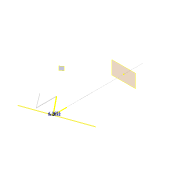
# Autodesk Inventor part: 00_Beampath_v0
Saved by Autodesk Inventor 2022 (Build 260153000, 153)
## iProperties
Created: 2022-04-09
Part Number: 00_Beampath_v0
Material: Generic
Document SubType Name: Modeling
Designer: Prakash Lab
Density: 1 g/cm^3
Appearance: Default
Author: Prakash Lab
Autodesk Inventor part; units mm, degrees
ref_plane "YZ Plane" through (0, 0, 0) normal (1, 0, 0) x (0, 1, 0)
ref_plane "XZ Plane" through (0, 0, 0) normal (0, 1, 0) x (-1, 0, 0)
ref_plane "XY Plane" through (0, 0, 0) normal (0, 0, 1) x (1, 0, 0)
ref_plane "Work Plane1" through (0, 0, 0) normal (0, 0, 1) x (1, 0, 0)
sketch "Sketch1" plane through (0, 0, 0) normal (0, 0, 1) x (1, 0, 0)
  circle A0 centre (0, 0) radius 0.5
  dimension "d0" = 1
  constraints: 1 centre point, 1 coincident
  measures "d0" diameter of A0
extrude "Extrusion1" add sketch "Sketch1" along normal blind 170 and the other way blind 105
sketch "Sketch2" plane through (0, 0, 170) normal (0, 0, 1) x (1, 0, 0)
  circle A0 centre (0, 0) radius 0.5
  circle A1 centre (0, 0) radius 0.820825
  constraints: 1 centre point, 1 coincident
extrude "Extrusion2" add sketch "Sketch2" along normal blind 75 contours A0 | A1
sketch "Sketch3" plane through (0, 0, 245) normal (0, 0, 1) x (1, 0, 0)
  circle A0 centre (0, 0) radius 0.820825
  circle A1 centre (0, 0) radius 0.5
  circle A2 centre (0, 0) radius 0.5
  constraints: 1 centre point, 1 coincident
extrude "Extrusion3" add sketch "Sketch3" along normal blind 75 contours A1
sketch "Sketch4" plane through (0, 0, 320) normal (0, 0, 1) x (1, 0, 0)
  circle A0 centre (0, 0) radius 0.820825
extrude "Extrusion4" add sketch "Sketch4" along normal blind 75
sketch "Sketch5" plane through (0, 0, 0) normal (0, 1, 0) x (-1, 0, 0)
  line L0 (-0.820825, 320) -> (-0.820825, 395)
  line L1 (-0.820825, 320) -> (-0.820825, 395)
  line L2 (0.820825, 320) -> (0.820825, 395)
  line L3 (0.820825, 395) -> (-0.820825, 395)
  line L4 (0, 395) -> (201.982812, 145.572)
  line L5 (0, 395) -> (-0.820825, 394.335309)
  line L6 (-0.820825, 394.335309) -> (80.573337, 293.82189)
  line L7 (80.573337, 293.82189) -> (81.394162, 294.486581)
  point P0 (0, 0)
  point P1 (0.820825, 393.986366)
  point P2 (0.820825, 392.308042)
  dimension "d11" = 39
  dimension "d12" = 249.428
  constraints: 8 end point, 2 point on line, 1 midpoint, 1 parallel, 1 perpendicular
  measures "d11" angle of L0 L4
  measures "d12" vertical distance of L4.start L4.end
ref_plane "Work Plane2" through (-201.982812, 0, 145.572) normal (-0.6293204, 0, -0.777146) x (0, -1, 0)
revolve "Revolution1" add sketch "Sketch5" angle 360 about axis through (0, 0, 395) along (-0.6293204, 0, -0.777146) contours L5 L4 L2 L6 | L2 L4 L7 L6
sketch "Sketch10" plane through (0, 0, 0) normal (0, 1, 0) x (-1, 0, 0)
  line L0 (82.214986, 295.151272) -> (80.573337, 293.82189)
  line L1 (82.214986, 295.151272) -> (80.573337, 293.82189)
  line L2 (81.394162, 294.486581) -> (81.394162, 406.830692)
  line L3 (82.214986, 295.151272) -> (79.881571, 295.151272)
  line L4 (79.881571, 295.151272) -> (79.881571, 406.830692)
  line L5 (79.881571, 406.830692) -> (81.394162, 406.830692)
  line L6 (82.214986, 295.151272) -> (0.820825, 395.664691)
  point P0 (0, 0)
  point P1 (2.462474, 393.637423)
  point P2 (79.881571, 298.0328)
  point P3 (81.394162, 296.164905)
  point P4 (81.394162, 295.151272)
  dimension "d18" = 39
  constraints: 8 end point, 2 perpendicular, 1 midpoint, 1 parallel
  measures "d18" angle of L6 L2
revolve "Revolution2" add sketch "Sketch10" angle 360 about axis through (-81.394162, 0, 294.486581) along (0, 0, 1) contours L3 L4 L6 L2 | L6 L4 L5 L2
sketch "Sketch11" plane through (0, 0, 0) normal (0, 1, 0) x (-1, 0, 0)
  line L0 (79.881571, 298.0328) -> (79.881571, 406.830692)
  line L1 (82.906753, 295.151272) -> (82.906753, 406.830692)
  line L2 (82.906753, 406.830692) -> (79.881571, 406.830692)
  line L3 (81.394162, 406.830692) -> (140.440427, 328.159447)
  line L4 (140.440427, 328.159447) -> (139.422813, 327.395682)
  line L5 (139.422813, 327.395682) -> (80.376547, 406.066927)
  line L6 (80.376547, 406.066927) -> (81.394162, 406.830692)
  point P0 (0, 0)
  constraints: 8 end point, 3 perpendicular, 1 midpoint, 1 point on line
revolve "Revolution3" add sketch "Sketch11" angle 360 about axis through (-81.394162, 0, 406.830692) along (-0.6002786, 0, -0.7997909) contours L5 L6 L3 L1 | L1 L3 L4 L5
sketch "Sketch12" plane through (0, 0, 0) normal (0, 1, 0) x (-1, 0, 0)
  line L0 (82.214986, 295.151272) -> (80.573337, 293.82189)
  line L1 (82.214986, 295.151272) -> (80.196137, 295.151272)
  line L2 (80.196137, 295.151272) -> (82.214986, 295.151272)
  line L3 (0.820825, 320) -> (-0.820825, 320)
  line L4 (4.715038, 389.177413) -> (-3.452339, 399.263283)
  line L5 (0, 383.095672) -> (0, 396.614396)
  line L6 (-2.252032, 394.202514) -> (2.252032, 395.797486)
  line L7 (79.881571, 298.0328) -> (0.820825, 395.664691)
  line L8 (-0.820825, 320) -> (-0.820825, 394.335309)
  line L9 (0.820825, 320) -> (0.820825, 392.308042)
  line L10 (80.573337, 293.82189) -> (0.820825, 392.308042)
  line L11 (-0.820825, 394.335309) -> (0, 395)
  line L12 (0, 395) -> (-0.820825, 394.335309)
  point P0 (0, 0)
  point P1 (0.820825, 392.308042)
  point P2 (2.462474, 393.637423)
  point P3 (0.820825, 392.308042)
  point P4 (0.820825, 393.986366)
  point P5 (0.820825, 395)
  point P6 (-0.820825, 395)
  point P7 (0, 395)
  dimension "d21" = 1.64165
  dimension "d22" = 0.82082
  constraints: 6 end point, 1 midpoint, 1 parallel, 1 vertical, 3 other
  measures "d21" distance between parallel lines of L9 L8
  measures "d22" distance between parallel lines of L8 L5
ref_plane "Work Plane5" through (0, 0, 395) normal (0.3338069, 0, 0.9426415) x (0, 1, 0)
sketch "Sketch13" plane through (0, 0, 395) normal (0.3338069, 0, 0.9426415) x (0, 1, 0)
  ellipse E0 centre (0, 0) end of major axis (1.056204, 0) minor radius 0.995622
  circle A0 centre (0, 0) radius 1.898257
  point P0 (0, -131.853709)
  point P1 (0, -0.995622)
  constraints: 1 centre point, 1 coincident, 1 vertical alignment
extrude "Extrusion7" cut sketch "Sketch13" along normal blind 25.4 contours E0 | A0
sketch "Sketch14" plane through (0, 0, 395) normal (0.3338069, 0, 0.9426415) x (0.9426415, 0, -0.3338069)
  ellipse E0 centre (0, 0) end of major axis (1.120472, 0) minor radius 1.056204 (0, 1.056204) -> (0, -1.056204) ccw
  line L0 (0, -0.820825) -> (0, -1.056204)
  ellipse E1 centre (0, 0) end of major axis (0.870771, 0) minor radius 0.820825 (0, -0.820825) -> (0, 0.820825) ccw
  line L1 (0, 1.056204) -> (0, 0.820825)
  circle A0 centre (0, 0) radius 0.310652
  point P0 (131.853709, 0)
  constraints: 1 centre point, 1 coincident, 2 other
extrude "Extrusion8" cut sketch "Sketch14" against normal blind 25.4 contours A0
sketch "Sketch15" plane through (0, 0, 0) normal (0, 1, 0) x (-1, 0, 0)
  line L0 (79.881571, 298.0328) -> (79.881571, 406.830692)
  line L1 (82.906753, 295.151272) -> (82.906753, 402.695767)
  line L2 (75.780569, 301.41879) -> (84.581608, 290.550413)
  line L3 (81.394162, 304.987675) -> (81.394162, 291.424331)
  line L4 (80.573337, 293.82189) -> (0.820825, 392.308042)
  line L5 (79.881571, 298.0328) -> (0.820825, 395.664691)
  line L6 (76.652956, 292.807632) -> (85.693899, 296.009198)
  line L7 (79.881571, 293.950944) -> (83.678666, 295.295566)
  line L8 (83.678666, 295.295566) -> (83.56271, 295.623018)
  line L9 (83.56271, 295.623018) -> (79.765614, 294.278396)
  line L10 (79.765614, 294.278396) -> (79.881571, 293.950944)
  line L11 (82.756792, 406.830692) -> (82.756792, 406.830692)
  line L12 (80.196137, 295.151272) -> (80.196137, 295.151272)
  line L13 (82.756792, 406.830692) -> (81.394162, 406.830692)
  line L14 (81.394162, 406.830692) -> (82.756792, 406.830692)
  line L15 (81.394162, 406.830692) -> (81.394162, 406.830692)
  line L16 (141.458041, 328.923212) -> (139.422813, 327.395682)
  line L17 (139.422813, 327.395682) -> (82.906753, 402.695767)
  line L18 (141.458041, 328.923212) -> (82.411776, 407.594457)
  line L19 (79.881571, 298.0328) -> (79.881571, 406.830692)
  line L20 (82.906753, 295.151272) -> (82.906753, 402.695767)
  line L21 (81.394162, 394.279852) -> (81.394162, 413.621168)
  line L22 (86.59775, 399.897607) -> (77.597609, 411.889091)
  line L23 (78.065498, 405.720493) -> (84.224665, 407.774741)
  line L24 (84.224665, 407.774741) -> (84.614224, 406.606742)
  line L25 (84.614224, 406.606742) -> (78.455057, 404.552494)
  line L26 (78.455057, 404.552494) -> (78.065498, 405.720493)
  point P0 (0, 0)
  point P1 (81.394162, 294.486581)
  dimension "d27" = 2.11241
  dimension "d28" = 3.02518
  dimension "d29" = 1.0562
  dimension "d30" = 1.51259
  dimension "d31" = 39
  dimension "d32" = 109.5
  dimension "d38" = 36.8899
  dimension "d39" = 71.5551
  dimension "d40" = 1.51259
  dimension "d41" = 2.5447
  dimension "d42" = 1.27235
  constraints: 26 end point, 8 parallel, 8 point on line, 2 perpendicular, 1 vertical
  measures "d27" distance between parallel lines of L5 L4
  measures "d28" distance between parallel lines of L1 L0
  measures "d29" distance between parallel lines of L2 L5
  measures "d30" distance between parallel lines of L1 L3
  measures "d31" angle of L3 L2
  measures "d32" angle of L6 L2
  measures "d38" angle of L22 L21
  measures "d39" angle of L21 L23
  measures "d40" distance between parallel lines of L1 L21
  measures "d41" distance between parallel lines of L18 L17
  measures "d42" distance between parallel lines of L22 L18
extrude "Extrusion9" add sketch "Sketch15" along normal mid plane 4
sketch "Sketch16" plane through (-83.678666, -2, 295.295566) normal (-0.3338069, 0, -0.9426415) x (-0.9426415, 0, 0.3338069)
  point P0 (-177.450668, 2)
sketch "Sketch17" plane through (-83.678666, -2, 295.295566) normal (-0.3338069, 0, -0.9426415) x (-0.9426415, 0, 0.3338069)
  line L0 (-367.961441, 2) -> (168.673723, 2)
  line L1 (168.673723, 2) -> (-367.961441, 2)
  line L2 (-2.423513, 0.943796) -> (-2.423513, 3.056204)
  circle A0 centre (-2.423513, 2) radius 1
  point P0 (-177.450668, 2)
  dimension "d35" = 2
  constraints: 1 centre point, 1 coincident, 1 midpoint
  measures "d35" diameter of A0
extrude "Extrusion10" cut sketch "Sketch17" along normal mid plane 4
sketch "Sketch18" plane through (-78.065498, -2, 405.720493) normal (0.316393, 0, 0.9486282) x (0.9486282, 0, -0.316393)
  line L0 (0, 0) -> (0, 4)
  line L1 (-6.492709, 4) -> (0, 4)
  line L2 (-6.492709, 0) -> (-6.492709, 4)
  line L3 (0, 0) -> (-6.492709, 0)
  ellipse E0 centre (-3.508923, 2) end of major axis (-2.16767, 2) minor radius 1.272351 (-3.508923, 3.272351) -> (-3.508923, 0.727649) ccw
  line L4 (-3.508923, 3.512591) -> (-3.508923, 3.272351)
  ellipse E1 centre (-3.508923, 2) end of major axis (-1.91442, 2) minor radius 1.512591 (-3.508923, 0.487409) -> (-3.508923, 3.512591) ccw
  line L5 (-3.508923, 0.727649) -> (-3.508923, 0.487409)
  line L6 (478.119806, 2) -> (-152.407058, 2)
  ellipse E2 centre (-3.919578, 2) end of major axis (-2.578325, 2) minor radius 1.272351 (-3.961542, 3.271728) -> (-3.961542, 0.728272) ccw
  ellipse E3 centre (-34.630845, 2) end of major axis (-34.630845, 3.272351) minor radius 1.206988
  circle A0 centre (-3.508923, 2) radius 1.690981
  point P0 (202.422256, 2)
  constraints: 1 centre point, 1 coincident, 1 vertical alignment, 4 other
extrude "Extrusion11" cut sketch "Sketch18" along normal blind 254 and the other way blind 1 contours A0 L6 E0 L5 E1 | L6 E1 L4 E0 A0 | L6 E0 L4 E1 | E1 L5 E0 L6
equation "\"d22\" = 0.5 * d21"
equation "\"d29\" = 0.5 * d27"
equation "\"d30\" = 0.5 * d28"
equation "\"d40\" = d30"
equation "\"d42\" = 0.5 * d41"
body "Solid1"
